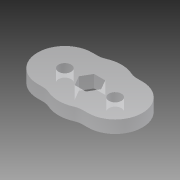
# Autodesk Inventor part: plastic_part_99
Saved by Autodesk Inventor 2013 (Build 170138000, 138)
## iProperties
Shininess: 20.0
Created: 2013-06-02
Part Number: plastic_part_99
Document SubType Name: Modeling
Designer: Noa Izumi
Material: Default
Density: 1 g/cm^3
Density: 0.0
Volumn: 0.0
Area: 0.0
PropertySet Name: Model Information
Control State: 0
Master: False
Checked Out: False
Author: Noa Izumi
Autodesk Inventor part; units mm, degrees
ref_plane "YZ Plane" through (0, 0, 0) normal (1, 0, 0) x (0, 1, 0)
ref_plane "XZ Plane" through (0, 0, 0) normal (0, 1, 0) x (-1, 0, 0)
ref_plane "XY Plane" through (0, 0, 0) normal (0, 0, 1) x (1, 0, 0)
sketch "Sketch1" plane through (0, 0, 0) normal (0, 0, 1) x (1, 0, 0)
  circle A0 centre (0, 0) radius 7.5
  arc A1 (6, -6.5) -> (6, 6.5) centre (6, 0) ccw
  line L0 (6, -6.5) -> (-6, -6.5)
  arc A2 (-6, 6.5) -> (-6, -6.5) centre (-6, 0) ccw
  line L1 (-6, 6.5) -> (6, 6.5)
  dimension "d0" = 15
  dimension "d6" = 6
  dimension "d8" = 6
  dimension "d22" = 6.5
  dimension "d23" = 6.5
  dimension "d24" = 12
  constraints: 4 end point, 4 point on circle, 3 centre point, 1 parallel
  measures "d0" diameter of A0
  measures "d6" distance of A1.centre A0.centre
  measures "d8" distance of A0.centre A2.centre
  measures "d22" radius of A1
  measures "d23" radius of A2
  measures "d24" distance of L1.start L1.end
extrude "Extrusion1" add sketch "Sketch1" along normal blind 3
sketch "草圖4" plane through (0, 0, 3) normal (0, 0, 1) x (1, 0, 0)
  arc A0 (3.7417, 6.5) -> (-3.7417, 6.5) centre (0, 0) ccw projected
  line L0 (1.3279, 2.3) -> (2.6558, 0)
  line L1 (2.6558, 0) -> (1.3279, -2.3)
  line L2 (1.3279, -2.3) -> (-1.3279, -2.3)
  line L3 (-1.3279, -2.3) -> (-2.6558, 0)
  line L4 (-2.6558, 0) -> (-1.3279, 2.3)
  line L5 (-1.3279, 2.3) -> (1.3279, 2.3)
  point P0 (-2.7439, 4.7667)
  point P1 (2.7439, 4.7667)
  point P2 (-6, -4.5)
  point P3 (6, -4.5)
  dimension "d17" = 4.6
  constraints: 12 end point, 1 coincident, 14 other
  measures "d17" distance between parallel lines of L2 L5
extrude "擠出2" cut sketch "草圖4" against normal through all
fillet "圓角2" radius 4 4 edges at (3.7417, -6.5, 1.5) (-3.7417, -6.5, 1.5) (3.7417, 6.5, 1.5) (-3.7417, 6.5, 1.5)
sketch "草圖5" plane through (0, 0, 3) normal (0, 0, 1) x (1, 0, 0)
  arc A0 (6, -6.5) -> (6, 6.5) centre (6, 0) ccw projected
  arc A1 (-6, 6.5) -> (-6, -6.5) centre (-6, 0) ccw projected
  constraints: 2 coincident
hole "孔2" at (-6, 0, 3) at (6, 0, 3) direction (0, 0, -1) diameter 3 end through all
